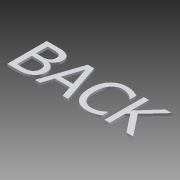
# Autodesk Inventor part: BackLabel
Saved by Autodesk Inventor 2012 (Build 160160000, 160)
## iProperties
Created: 2014-07-21
Part Number: BackLabel
Material: Default
Document SubType Name: Modeling
Designer: Anon
Density: 1 g/cm^3
Author: Anon
Autodesk Inventor part; units mm, degrees
ref_plane "YZ Plane" through (0, 0, 0) normal (1, 0, 0) x (0, 1, 0)
ref_plane "XZ Plane" through (0, 0, 0) normal (0, 1, 0) x (-1, 0, 0)
ref_plane "XY Plane" through (0, 0, 0) normal (0, 0, 1) x (1, 0, 0)
sketch "Sketch1" plane through (0, 0, 0) normal (0, 0, 1) x (1, 0, 0)
  line L0 (-14.2269, 7.3651) -> (16.5142, 7.3651) construction
  line L1 (16.5142, 7.3651) -> (16.5142, -10.6587) construction
  line L2 (16.5142, -10.6587) -> (-14.2269, -10.6587) construction
  line L3 (-14.2269, -10.6587) -> (-14.2269, 7.3651) construction
  spline S0 degree 2 poles (-11.4984, 4.8776) (-11.4984, 4.6167) (-11.6969, 4.2168) (-11.8614, 4.0863) knots 0 0 0 1 2 2 2
  spline S1 degree 2 poles (-11.8614, 4.0863) (-12.06, 3.9331) (-12.5109, 3.8027) (-12.8683, 3.8027) knots 0 0 0 1 2 2 2
  line L4 (-12.8683, 3.8027) -> (-13.8724, 3.8027)
  line L5 (-13.8724, 3.8027) -> (-13.8724, 7.3027)
  line L6 (-13.8724, 7.3027) -> (-12.9449, 7.3027)
  spline S2 degree 2 poles (-12.9449, 7.3027) (-12.5705, 7.3027) (-12.1961, 7.2544) (-12.0259, 7.1608) knots 0 0 0 1 2 2 2
  spline S3 degree 2 poles (-12.0259, 7.1608) (-11.8359, 7.0616) (-11.6629, 6.7354) (-11.6629, 6.5142) knots 0 0 0 1 2 2 2
  spline S4 degree 2 poles (-11.6629, 6.5142) (-11.6629, 6.2674) (-11.9238, 5.876) (-12.1536, 5.7654) knots 0 0 0 1 2 2 2
  line L7 (-12.1536, 5.7654) -> (-12.1536, 5.7484)
  spline S5 degree 2 poles (-12.1536, 5.7484) (-11.8416, 5.6633) (-11.4984, 5.2123) (-11.4984, 4.8776) knots 0 0 0 1 2 2 2
  spline S6 degree 2 poles (-11.9834, 4.8578) (-11.9834, 5.0563) (-12.0968, 5.3116) (-12.267, 5.4023) knots 0 0 0 1 2 2 2
  spline S7 degree 2 poles (-12.267, 5.4023) (-12.3776, 5.4591) (-12.6386, 5.4931) (-12.8797, 5.4931) knots 0 0 0 1 2 2 2
  line L8 (-12.8797, 5.4931) -> (-13.4072, 5.4931)
  line L9 (-13.4072, 5.4931) -> (-13.4072, 4.1997)
  line L10 (-13.4072, 4.1997) -> (-13.03, 4.1997)
  spline S8 degree 2 poles (-13.03, 4.1997) (-12.7237, 4.1997) (-12.372, 4.2565) (-12.2358, 4.3472) knots 0 0 0 1 2 2 2
  spline S9 degree 2 poles (-12.2358, 4.3472) (-12.1053, 4.4408) (-11.9834, 4.6734) (-11.9834, 4.8578) knots 0 0 0 1 2 2 2
  spline S10 degree 2 poles (-12.1479, 6.4489) (-12.1479, 6.5737) (-12.233, 6.7609) (-12.3266, 6.8148) knots 0 0 0 1 2 2 2
  spline S11 degree 2 poles (-12.3266, 6.8148) (-12.44, 6.8772) (-12.7151, 6.9056) (-12.9619, 6.9056) knots 0 0 0 1 2 2 2
  line L11 (-12.9619, 6.9056) -> (-13.4072, 6.9056)
  line L12 (-13.4072, 6.9056) -> (-13.4072, 5.8817)
  line L13 (-13.4072, 5.8817) -> (-12.8797, 5.8817)
  spline S12 degree 2 poles (-12.8797, 5.8817) (-12.6613, 5.8817) (-12.4542, 5.927) (-12.3436, 5.998) knots 0 0 0 1 2 2 2
  spline S13 degree 2 poles (-12.3436, 5.998) (-12.2358, 6.066) (-12.1479, 6.2844) (-12.1479, 6.4489) knots 0 0 0 1 2 2 2
  line L14 (-11.4133, 3.8027) -> (-10.2334, 7.3027)
  line L15 (-10.2334, 7.3027) -> (-9.6604, 7.3027)
  line L16 (-9.6604, 7.3027) -> (-8.4805, 3.8027)
  line L17 (-8.4805, 3.8027) -> (-8.9712, 3.8027)
  line L18 (-8.9712, 3.8027) -> (-9.2889, 4.7812)
  line L19 (-9.2889, 4.7812) -> (-10.6248, 4.7812)
  line L20 (-10.6248, 4.7812) -> (-10.9425, 3.8027)
  line L21 (-10.9425, 3.8027) -> (-11.4133, 3.8027)
  line L22 (-9.4165, 5.1783) -> (-9.9583, 6.8262)
  line L23 (-9.9583, 6.8262) -> (-10.4972, 5.1783)
  line L24 (-10.4972, 5.1783) -> (-9.4165, 5.1783)
  spline S14 degree 2 poles (-6.7816, 3.7403) (-7.122, 3.7403) (-7.6977, 3.97) (-7.9076, 4.1997) knots 0 0 0 1 2 2 2
  spline S15 degree 2 poles (-7.9076, 4.1997) (-8.1175, 4.4266) (-8.3472, 5.1074) (-8.3472, 5.5498) knots 0 0 0 1 2 2 2
  spline S16 degree 2 poles (-8.3472, 5.5498) (-8.3472, 5.9894) (-8.1232, 6.6418) (-7.9104, 6.8829) knots 0 0 0 1 2 2 2
  spline S17 degree 2 poles (-7.9104, 6.8829) (-7.7006, 7.1183) (-7.1276, 7.3651) (-6.7731, 7.3651) knots 0 0 0 1 2 2 2
  spline S18 degree 2 poles (-6.7731, 7.3651) (-6.5972, 7.3651) (-6.2881, 7.314) (-6.1576, 7.2743) knots 0 0 0 1 2 2 2
  spline S19 degree 2 poles (-6.1576, 7.2743) (-6.0442, 7.2374) (-5.8087, 7.1325) (-5.6925, 7.0701) knots 0 0 0 1 2 2 2
  line L25 (-5.6925, 7.0701) -> (-5.6925, 6.5085)
  line L26 (-5.6925, 6.5085) -> (-5.7293, 6.5085)
  spline S20 degree 2 poles (-5.7293, 6.5085) (-5.7917, 6.5652) (-5.9846, 6.724) (-6.1236, 6.8006) knots 0 0 0 1 2 2 2
  spline S21 degree 2 poles (-6.1236, 6.8006) (-6.2569, 6.8744) (-6.5717, 6.968) (-6.7759, 6.968) knots 0 0 0 1 2 2 2
  spline S22 degree 2 poles (-6.7759, 6.968) (-7, 6.968) (-7.3999, 6.7836) (-7.5502, 6.6078) knots 0 0 0 1 2 2 2
  spline S23 degree 2 poles (-7.5502, 6.6078) (-7.6977, 6.4291) (-7.8622, 5.8873) (-7.8622, 5.5498) knots 0 0 0 1 2 2 2
  spline S24 degree 2 poles (-7.8622, 5.5498) (-7.8622, 5.1896) (-7.6892, 4.6706) (-7.5389, 4.4919) knots 0 0 0 1 2 2 2
  spline S25 degree 2 poles (-7.5389, 4.4919) (-7.3914, 4.3189) (-6.9972, 4.143) (-6.7759, 4.143) knots 0 0 0 1 2 2 2
  spline S26 degree 2 poles (-6.7759, 4.143) (-6.5745, 4.143) (-6.2314, 4.2423) (-6.098, 4.316) knots 0 0 0 1 2 2 2
  spline S27 degree 2 poles (-6.098, 4.316) (-5.9704, 4.3898) (-5.7804, 4.5429) (-5.7265, 4.5968) knots 0 0 0 1 2 2 2
  line L27 (-5.7265, 4.5968) -> (-5.6925, 4.5968)
  line L28 (-5.6925, 4.5968) -> (-5.6925, 4.0409)
  spline S28 degree 2 poles (-5.6925, 4.0409) (-5.8087, 3.987) (-6.013, 3.8877) (-6.1576, 3.8424) knots 0 0 0 1 2 2 2
  spline S29 degree 2 poles (-6.1576, 3.8424) (-6.3108, 3.7913) (-6.5717, 3.7403) (-6.7816, 3.7403) knots 0 0 0 1 2 2 2
  line L29 (-2.7058, 3.8027) -> (-3.31, 3.8027)
  line L30 (-3.31, 3.8027) -> (-4.5891, 5.4307)
  line L31 (-4.5891, 5.4307) -> (-4.7933, 5.2009)
  line L32 (-4.7933, 5.2009) -> (-4.7933, 3.8027)
  line L33 (-4.7933, 3.8027) -> (-5.2585, 3.8027)
  line L34 (-5.2585, 3.8027) -> (-5.2585, 7.3027)
  line L35 (-5.2585, 7.3027) -> (-4.7933, 7.3027)
  line L36 (-4.7933, 7.3027) -> (-4.7933, 5.6945)
  line L37 (-4.7933, 5.6945) -> (-3.3582, 7.3027)
  line L38 (-3.3582, 7.3027) -> (-2.7909, 7.3027)
  line L39 (-2.7909, 7.3027) -> (-4.2403, 5.7398)
  line L40 (-4.2403, 5.7398) -> (-2.7058, 3.8027)
  point P0 (0, 0)
  constraints: 2 other
extrude "BackLabel" add sketch "Sketch1" along normal blind 0.2
body "Solid1"
